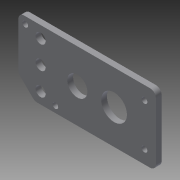
# Autodesk Inventor part: Granny Gearbox Output Plate
Saved by Autodesk Inventor 2015 (Build 190159000, 159)
## iProperties
Created: 2016-02-25
Part Number: Granny Gearbox Output Plate
Material: Generic
Document SubType Name: Modeling
Designer: sethbattis
Density: 1 g/cm^3
Appearance: Default
Author: sethbattis
Autodesk Inventor part; units mm, degrees
ref_plane "YZ Plane" through (0, 0, 0) normal (1, 0, 0) x (0, 1, 0)
ref_plane "XZ Plane" through (0, 0, 0) normal (0, 1, 0) x (-1, 0, 0)
ref_plane "XY Plane" through (0, 0, 0) normal (0, 0, 1) x (1, 0, 0)
sketch "Shaft Alignment" plane through (0, 0, 0) normal (0, 0, 1) x (1, 0, 0)
  circle A0 centre (40.6908, 0) radius 14.2875
  circle A1 centre (0, 0) radius 11.1125
  circle A2 centre (-40.7035, -0.0359) radius 5.5626
  line L0 (11.1125, 0) -> (11.1125, 11.8355) construction
  line L1 (26.4033, 0) -> (26.4033, 12.8304) construction
  circle A3 centre (-40.7035, 25.3641) radius 5.5626
  circle A4 centre (-40.7035, -25.4359) radius 5.5626
  line L2 (-40.7035, -0.0359) -> (0, 0) construction
  line L3 (0, 0) -> (40.6908, 0) construction
  line L4 (-40.7035, 25.3641) -> (-40.7035, -25.4359) construction
  line L5 (-46.2661, 25.3641) -> (-46.2661, -25.4359) construction
  line L6 (-40.7035, -5.5985) -> (-46.2661, -5.5985) construction
  line L7 (-40.7035, -19.8733) -> (-46.2661, -19.8733) construction
  line L8 (-40.7035, 19.8015) -> (-46.2661, 19.8015) construction
  line L9 (-40.7035, 5.5267) -> (-46.2661, 5.5267) construction
  line L10 (-40.7035, -5.5985) -> (-0.0001, -11.1125) construction
  line L11 (-35.1409, -0.031) -> (-35.1353, -6.3528) construction
  line L12 (-11.1125, -0.0098) -> (-11.104, -9.6083) construction
  line L13 (0, 11.1125) -> (43.74, 13.9583) construction
  point P0 (-33.5787, -27.5177)
  dimension "d0" = 28.575
  dimension "d1" = 22.225
  dimension "d2" = 11.1252
  dimension "d3" = 15.2908
  dimension "d12" = 14.2748
  dimension "d13" = 14.2748
  dimension "d14" = 24.0284
  constraints: 28 end point, 16 point on line, 10 point on circle, 7 tangent, 4 centre point, 4 perpendicular, 3 parallel, 2 coincident, 2 equal radius, 2 vertical, 1 midpoint, 3 other
  measures "d1" diameter of A1
  measures "d2" diameter of A2
  measures "d3" distance between parallel lines of L1 L0
  measures "d12" distance between parallel lines of L7 L6
  measures "d13" distance between parallel lines of L9 L8
  measures "d14" distance between parallel lines of L12 L11
sketch "Gear Shadows" plane through (0, 0, 0) normal (0, 0, 1) x (1, 0, 0)
  circle A0 centre (-40.7035, -0.0359) radius 5.5626 projected
  circle A1 centre (0, 0) radius 11.1125 projected
  circle A2 centre (40.6908, 0) radius 14.2875 projected
  circle A3 centre (40.6908, 0) radius 33.02 construction
  circle A4 centre (0, 0) radius 33.02 construction
  circle A5 centre (40.6908, 0) radius 36.195 construction
  circle A6 centre (0, 0) radius 36.195 construction
  circle A7 centre (-40.7035, -0.0359) radius 10.1854 construction
  circle A8 centre (-40.7035, -0.0359) radius 31.75 construction
  dimension "d32" = 66.04
  dimension "d33" = 72.39
  dimension "d34" = 20.3708
  dimension "d35" = 63.5
  constraints: 6 centre point, 6 coincident, 2 equal radius, 6 other
  measures "d32" diameter of A3
  measures "d33" diameter of A5
  measures "d34" diameter of A7
  measures "d35" diameter of A8
sketch "Existing Mounting Holes" plane through (0, 0, 0) normal (0, 0, 1) x (1, 0, 0)
  circle A0 centre (-39.9633, 23.3553) radius 2.5527 construction
  circle A1 centre (-39.9633, -23.3553) radius 2.5527 construction
  circle A2 centre (74.3367, -23.3553) radius 2.5527 construction
  circle A3 centre (74.3367, 23.3553) radius 2.5527 construction
  line L0 (-46.3133, 29.7053) -> (80.6867, 29.7053) construction
  line L1 (80.6867, 29.7053) -> (80.6867, -29.7053) construction
  line L2 (80.6867, -29.7053) -> (-46.3133, -29.7053) construction
  line L3 (-46.3133, -29.7053) -> (-46.3133, 29.7053) construction
  line L4 (-39.9633, 23.3553) -> (74.3367, 23.3553) construction
  line L5 (74.3367, 23.3553) -> (74.3367, -23.3553) construction
  line L6 (74.3367, -23.3553) -> (-39.9633, -23.3553) construction
  line L7 (-39.9633, -23.3553) -> (-39.9633, 23.3553) construction
  line L8 (-65.3633, 38.1) -> (87.0367, 38.1) construction
  line L9 (87.0367, 38.1) -> (87.0367, -38.1) construction
  line L10 (87.0367, -38.1) -> (-65.3633, -38.1) construction
  line L11 (-65.3633, -38.1) -> (-65.3633, 38.1) construction
  line L12 (-65.3633, 0) -> (87.0367, 0) construction
  circle A4 centre (40.6908, 0) radius 36.195 construction
  circle A5 centre (74.3367, 23.3553) radius 4.7625 construction
  circle A6 centre (74.3367, -23.3553) radius 4.7625 construction
  circle A7 centre (-39.9633, -23.3553) radius 4.7625 construction
  circle A8 centre (-39.9633, 23.3553) radius 4.7625 construction
  point P0 (0, 0)
  dimension "d19" = 127
  dimension "d20" = 59.4106
  dimension "d21" = 6.35
  dimension "d22" = 6.35
  dimension "d23" = 6.35
  dimension "d24" = 6.35
  dimension "d25" = 152.4
  dimension "d26" = 76.2
  dimension "d27" = 5.1054
  dimension "d30" = 12.7
  dimension "d40" = 9.525
  constraints: 26 end point, 8 centre point, 8 coincident, 6 equal radius, 6 horizontal, 6 parallel, 4 perpendicular, 2 midpoint, 2 tangent, 2 other
  measures "d19" distance of L0.start L0.end
  measures "d20" distance of L0.end L1.end
  measures "d21" distance between parallel lines of L4 L0
  measures "d22" distance between parallel lines of L3 L7
  measures "d23" distance between parallel lines of L2 L6
  measures "d24" distance between parallel lines of L5 L1
  measures "d25" distance of L8.start L8.end
  measures "d26" distance of L10.end L8.start
  measures "d27" diameter of A0
  measures "d30" distance between parallel lines of L9 L5
  measures "d40" diameter of A5
sketch "New Mounting Holes" plane through (0, 0, 0) normal (0, 0, 1) x (1, 0, 0)
  circle A0 centre (74.3367, 23.3553) radius 3.175
  circle A1 centre (74.3367, -23.3553) radius 3.175
  circle A2 centre (-57.7242, 30.4609) radius 3.175
  circle A3 centre (-24.3812, -30.912) radius 3.175
  line L0 (-65.3633, -38.1) -> (-65.3633, 38.1) construction
  line L1 (87.0367, -38.1) -> (-65.3633, -38.1) construction
  line L2 (87.0367, 38.1) -> (87.0367, -38.1) construction
  line L3 (-65.3633, 38.1) -> (87.0367, 38.1) construction
  line L4 (-55.8383, 38.1) -> (-55.8383, -38.1) construction
  line L5 (-65.3633, 28.575) -> (87.0367, 28.575) construction
  line L6 (-65.3633, -28.575) -> (87.0367, -28.575) construction
  line L7 (77.5117, 38.1) -> (77.5117, -38.1) construction
  circle A4 centre (-40.7035, -0.0359) radius 31.75 construction
  circle A5 centre (40.6908, 0) radius 36.195 construction
  circle A6 centre (0, 0) radius 36.195 construction
  line L8 (-57.7242, 30.4609) -> (-55.8383, 30.4609) construction
  line L9 (-57.7242, 30.4609) -> (-57.7242, 28.575) construction
  dimension "d31" = 6.35
  dimension "d36" = 9.525
  dimension "d37" = 9.525
  dimension "d38" = 9.525
  dimension "d39" = 9.525
  constraints: 12 end point, 10 point on line, 6 perpendicular, 4 centre point, 3 equal radius, 3 tangent, 2 coincident, 1 vertical, 4 other
  measures "d31" diameter of A0
  measures "d36" distance between parallel lines of L1 L6
  measures "d37" distance between parallel lines of L0 L4
  measures "d38" distance between parallel lines of L3 L5
  measures "d39" distance between parallel lines of L2 L7
sketch "Labels" plane through (0, 0, 0) normal (0, 0, 1) x (1, 0, 0)
  circle A0 centre (-40.7035, -0.0359) radius 5.5626 projected
  circle A1 centre (-40.7035, 25.3641) radius 5.5626 projected
  circle A2 centre (-40.7035, -25.4359) radius 5.5626 projected
  circle A3 centre (0, 0) radius 11.1125 projected
  circle A4 centre (40.6908, 0) radius 14.2875 projected
  line L0 (-5.8677, 26.2224) -> (48.5566, 26.2224) construction
  line L1 (48.5566, 26.2224) -> (48.5566, 22.1963) construction
  line L2 (48.5566, 22.1963) -> (-5.8677, 22.1963) construction
  line L3 (-5.8677, 22.1963) -> (-5.8677, 26.2224) construction
  constraints: 7 other
sketch "Exterior" plane through (0, 0, 0) normal (0, 0, 1) x (1, 0, 0)
  line L0 (-59.0133, 38.1) -> (80.6867, 38.1)
  line L1 (87.0367, 31.75) -> (87.0367, -31.75)
  line L2 (80.6867, -38.1) -> (-44.6678, -38.1)
  arc A0 (87.0367, 31.75) -> (80.6867, 38.1) centre (80.6867, 31.75) ccw
  arc A1 (80.6867, -38.1) -> (87.0367, -31.75) centre (80.6867, -31.75) ccw
  arc A2 (-59.0133, 38.1) -> (-65.3633, 31.75) centre (-59.0133, 31.75) ccw
  circle A3 centre (-40.7035, -0.0359) radius 31.75 construction
  line L3 (-65.3633, -17.4045) -> (-65.3633, 31.75)
  line L4 (-63.5034, -21.8946) -> (-49.1579, -36.2401)
  line L5 (-65.3633, -38.1) -> (-65.3633, 38.1) construction
  line L6 (87.0367, -38.1) -> (-65.3633, -38.1) construction
  arc A4 (-49.1579, -36.2401) -> (-44.6678, -38.1) centre (-44.6678, -31.75) ccw
  arc A5 (-65.3633, -17.4045) -> (-63.5034, -21.8946) centre (-59.0133, -17.4045) ccw
  point P0 (87.0367, 38.1)
  point P1 (-65.3633, -20.0348)
  point P2 (-47.2981, -38.1)
  dimension "d41" = 6.35
  dimension "d42" = 6.35
  dimension "d46" = 45
  dimension "d47" = 6.35
  constraints: 10 end point, 10 point on circle, 10 tangent, 9 point on line, 5 centre point, 2 equal radius, 2 parallel, 1 horizontal, 1 perpendicular, 2 other
  measures "d41" radius of A0
  measures "d42" radius of A1
  measures "d46" angle of L4 L5
  measures "d47" radius of A4
extrude "Extrusion1" add sketch "Exterior" against normal blind 6.35
extrude "Extrusion2" cut sketch "New Mounting Holes" against normal through all
extrude "Extrusion3" cut sketch "Labels" against normal through all
equation "\"d12\" = d13"
equation "\"d22\" = d21"
equation "\"d23\" = d21"
equation "\"d24\" = d21"
body "Solid1"
